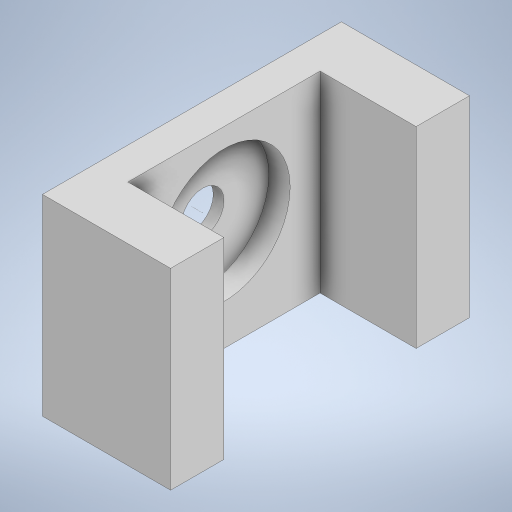
# Autodesk Inventor part: holdervegg
Saved by Autodesk Inventor 2023 (Build 270158000, 158)
## iProperties
Created: 2023-04-03
Part Number: holdervegg
Material: Generic
Document SubType Name: Modeling
Designer: Markus
Density: 1 g/cm^3
Appearance: Default
Author: Markus
Autodesk Inventor part; units mm, degrees
ref_plane "YZ Plane" through (0, 0, 0) normal (1, 0, 0) x (0, 1, 0)
ref_plane "XZ Plane" through (0, 0, 0) normal (0, 1, 0) x (-1, 0, 0)
ref_plane "XY Plane" through (0, 0, 0) normal (0, 0, 1) x (1, 0, 0)
sketch "Sketch1" plane through (0, 0, 0) normal (1, 0, 0) x (0, 1, 0)
  line L0 (0, 0) -> (18, 0)
  line L1 (18, 0) -> (18, -20)
  line L2 (18, -20) -> (0, -20)
  line L3 (0, -20) -> (0, 0)
  dimension "d0" = 18
  dimension "d1" = 20
  constraints: 8 end point, 2 parallel, 1 horizontal, 1 perpendicular
  measures "d0" distance of L1.end L2.end
  measures "d1" distance of L0.end L1.end
extrude "Extrusion1" add sketch "Sketch1" along normal blind 3
sketch "Sketch2" plane through (3, 0, 0) normal (1, 0, 0) x (0, 0, -1)
  line L0 (0, 0) -> (20, 0) projected
  line L1 (20, 18) -> (0, 18) projected
  line L2 (0, 0) -> (1, 0)
  line L3 (1, 0) -> (1, 18)
  line L4 (1, 18) -> (0, 18)
  line L5 (0, 18) -> (0, 0)
  line L6 (20, 0) -> (20, 18) projected
  line L7 (20, 0) -> (19, 0)
  line L8 (19, 0) -> (19, 18)
  line L9 (19, 18) -> (20, 18)
  line L10 (20, 18) -> (20, 0)
  dimension "d4" = 1
  dimension "d5" = 1
  constraints: 16 end point, 4 parallel, 2 horizontal, 2 perpendicular, 2 point on line
  measures "d4" distance of L4.end L3.end
  measures "d5" distance of L8.end L9.end
extrude "Extrusion2" add sketch "Sketch2" along normal blind 5 contours L5 L1 L3 L0 | L8 L1 L6 L0
sketch "Sketch3" plane through (3, 0, 0) normal (1, 0, 0) x (0, 0, -1)
  circle A0 centre (10, 10) radius 0.009
  circle A1 centre (10, 10) radius 2
  point P0 (0, 0)
  dimension "d8" = 4
  constraints: 2 centre point, 1 coincident
  measures "d8" diameter of A1
extrude "Extrusion3" cut sketch "Sketch3" against normal blind 5
sketch "Sketch4" plane through (0, 0, 0) normal (0, 0, 1) x (1, 0, 0)
  line L0 (0, 0) -> (8, 0)
  line L1 (8, 0) -> (8, 18)
  line L2 (8, 18) -> (0, 18)
  line L3 (0, 18) -> (0, 0)
  constraints: 8 end point, 2 parallel, 1 horizontal, 1 perpendicular
extrude "Extrusion4" add sketch "Sketch4" along normal blind 4
sketch "Sketch5" plane through (0, 0, -20) normal (0, 0, -1) x (-1, 0, 0)
  line L0 (0, 18) -> (0, 0) projected
  line L1 (-8, 0) -> (-8, 18) projected
  line L2 (0, 18) -> (-8, 18)
  line L3 (-8, 18) -> (-8, 0)
  line L4 (-8, 0) -> (0, 0)
  line L5 (0, 0) -> (0, 18)
  constraints: 8 end point, 2 parallel, 1 horizontal, 1 perpendicular
extrude "Extrusion5" add sketch "Sketch5" along normal blind 4
sketch "Sketch6" plane through (8, 0, 0) normal (1, 0, 0) x (0, 0, -1)
  line L0 (19, 0) -> (24, 0) projected
  line L1 (24, 0) -> (19, 0)
  line L2 (19, 0) -> (19, 18)
  line L3 (19, 18) -> (24, 18)
  line L4 (24, 18) -> (24, 0)
  line L5 (1, 0) -> (-4, 0) projected
  line L6 (1, 0) -> (1, 18) projected
  line L7 (-4, 0) -> (1, 0)
  line L8 (1, 0) -> (1, 18)
  line L9 (1, 18) -> (-4, 18)
  line L10 (-4, 18) -> (-4, 0)
  point P0 (0, 0)
  constraints: 16 end point, 4 parallel, 2 horizontal, 2 perpendicular
extrude "Extrusion6" add sketch "Sketch6" along normal blind 4
sketch "Sketch7" plane through (3, 0, 0) normal (1, 0, 0) x (0, 0, -1)
  circle A0 centre (10, 10) radius 0.009 projected
  circle A1 centre (10, 10) radius 6
  point P0 (0, 0)
  dimension "d17" = 12
  constraints: 1 centre point, 1 coincident
  measures "d17" diameter of A1
extrude "Extrusion7" cut sketch "Sketch7" against normal blind 2
sketch "Sketch8" plane through (3, 0, 0) normal (1, 0, 0) x (0, 0, -1)
  circle A0 centre (10, 10) radius 0.009 projected
  circle A1 centre (10, 10) radius 6.2
  point P0 (0, 0)
  dimension "d20" = 12.4
  constraints: 1 centre point, 1 coincident
  measures "d20" diameter of A1
extrude "Extrusion8" cut sketch "Sketch8" against normal blind 2 contours A0 | A1
body "Solid1"
